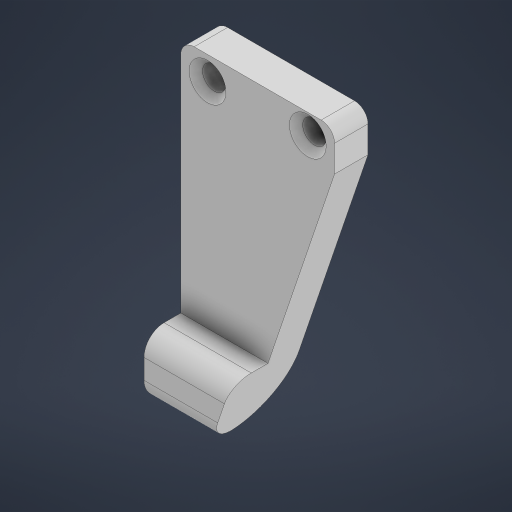
# Autodesk Inventor part: Lupfer Seite
Saved by Autodesk Inventor 2024.2 (Build 282272000, 272)
## iProperties
Created: 2023-12-02
Part Number: Lupfer Seite
Material: Generisch
Document SubType Name: Modeling
Designer: jacob
Density: 1 g/cm^3
Appearance: Vorgabe
Author: jacob
Autodesk Inventor part; units mm, degrees
ref_plane "YZ Plane" through (0, 0, 0) normal (1, 0, 0) x (0, 1, 0)
ref_plane "XZ Plane" through (0, 0, 0) normal (0, 1, 0) x (-1, 0, 0)
ref_plane "XY Plane" through (0, 0, 0) normal (0, 0, 1) x (1, 0, 0)
sketch "Skizze1" plane through (0, 0, 0) normal (0, 0, 1) x (1, 0, 0)
  line L0 (10, 0) -> (23, 38.5)
  line L1 (23, 38.5) -> (23, 44.5)
  line L2 (23, 44.5) -> (0, 44.5)
  line L3 (0, 44.5) -> (0, 0)
  line L4 (10, 0) -> (0, 0)
  dimension "d0" = 38.5
  dimension "d1" = 6
  dimension "d2" = 23
  dimension "d4" = 10
  constraints: 10 end point, 2 perpendicular, 1 coincident, 1 horizontal, 1 vertical alignment
  measures "d0" vertical distance of L0.start L0.end
  measures "d1" distance of L0.end L1.end
  measures "d2" distance of L1.end L2.end
  measures "d4" distance of L0.start L3.end
extrude "Extrusion1" add sketch "Skizze1" along normal blind 5
sketch "Skizze3" plane through (0, 0, 5) normal (0, 0, 1) x (1, 0, 0)
  line L0 (23, 38.5) -> (23, 44.5) projected
  line L1 (23, 41.5) -> (18.9958, 41.5) construction
  line L2 (4.0042, 41) -> (0, 41) construction
  line L3 (0, 44.5) -> (0, 0) construction
  dimension "d35" = 0.5
  dimension "d36" = 15
  constraints: 4 end point, 2 horizontal, 1 horizontal alignment, 1 midpoint, 1 parallel, 1 point on line
  measures "d35" distance between parallel lines of L1 L2
  measures "d36" distance of L1.end L2.start
hole "Bohrung2" at (4.0042, 41, 5) at (18.9958, 41.5, 5) direction (0, 0, -1) diameter 3.5 end through all
sketch "Skizze4" plane through (0, 0, 5) normal (0, 0, 1) x (1, 0, 0)
  line L0 (0, 44.5) -> (0, 0) projected
  line L1 (0, 9) -> (13.039, 9)
  line L2 (0, 0) -> (10, 0) projected
  line L3 (10, 0) -> (23, 38.5) projected
  dimension "d24" = 9
  constraints: 2 end point, 2 point on line, 1 horizontal
  measures "d24" distance between parallel lines of L2 L1
extrude "Extrusion2" add sketch "Skizze4" along normal blind 5.5
sketch "Skizze2" plane through (0, 0, 0) normal (-1, 0, 0) x (0, 0, 1)
  line L0 (0, 0) -> (5, 0) projected
  line L1 (5, 9) -> (10.5, 9) projected
  line L2 (10.5, 9) -> (10.5, 0) projected
  point P0 (7.5, 3.5)
  dimension "d27" = 3.5
  dimension "d37" = 3
  measures "d27" vertical distance of L2.end point (7.5, 3.5)
  measures "d37" distance from line of L2 point (7.5, 3.5)
hole "Bohrung1" at (0, 3.5, 7.5) direction (1, 0, 0) diameter 4.3 depth 8
fillet "Rundung2" radius 8 1 edges at (5, 0, 0)
fillet "Rundung3" radius 3 1 edges at (6.5195, 9, 10.5)
fillet "Rundung4" radius 3 1 edges at (5, 0, 10.5)
chamfer "Fasen1" distance 1 angle 45 2 edges at (4.0042, 42.75, 5) (18.9958, 43.25, 5)
fillet "Rundung5" radius 2 2 edges at (0, 44.5, 2.5) (23, 44.5, 2.5)
